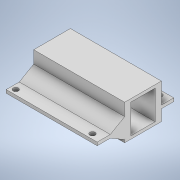
# Autodesk Inventor part: U2D2 Plate
Saved by Autodesk Inventor 2022 (Build 260153000, 153)
## iProperties
Created: 2021-09-20
Part Number: U2D2 Plate
Material: Generic
Document SubType Name: Modeling
Designer: kylem
Density: 1 g/cm^3
Appearance: Default
Author: kylem
Autodesk Inventor part; units mm, degrees
ref_plane "YZ Plane" through (0, 0, 0) normal (1, 0, 0) x (0, 1, 0)
ref_plane "XZ Plane" through (0, 0, 0) normal (0, 1, 0) x (-1, 0, 0)
sketch "Sketch1" plane through (0, 0, 0) normal (0, 1, 0) x (-1, 0, 0)
  line L0 (0, 0) -> (3, 0)
  line L1 (3, 0) -> (3, -3)
  line L2 (0, 0) -> (-48.04, 0)
  line L3 (-48.04, 0) -> (-54, 0)
  line L4 (3, -3) -> (-54, -3)
  line L5 (-54, -3) -> (-54, 45)
  line L6 (-54, 45) -> (3, 45)
  line L7 (3, 45) -> (3, -3)
  line L8 (3, 21) -> (6.1215, 21)
  circle A0 centre (0, 0) radius 1.65
  circle A1 centre (-48.04, 0) radius 1.65
  line L9 (0, 42) -> (-48.04, 42)
  circle A2 centre (0, 42) radius 1.65
  circle A3 centre (-48.04, 42) radius 1.65
  line L10 (-54, -3) -> (-54, 8.785)
  line L11 (-54, 8.785) -> (-9.9, 8.785)
  line L12 (-9.9, 8.785) -> (-9.9, 23.785)
  line L13 (-9.9, 23.785) -> (-54, 23.785)
  dimension "d0" = 3
  dimension "d1" = 3
  dimension "d2" = 48.04
  dimension "d3" = 5.96
  dimension "d4" = 48
  dimension "d5" = 3.3
  dimension "d6" = 3.3
  dimension "d7" = 11.785
  dimension "d8" = 44.1
  dimension "d9" = 15
  constraints: 28 end point, 5 perpendicular, 4 centre point, 4 coincident, 4 horizontal, 4 symmetric about line, 3 point on line, 2 parallel, 1 midpoint, 2 other
  measures "d0" distance of L0.start L0.end
  measures "d1" distance of L0.end L1.end
  measures "d2" distance of L0.start L2.end
  measures "d3" distance of L2.end L3.end
  measures "d4" distance of L4.end L5.end
  measures "d5" diameter of A0
  measures "d6" diameter of A1
  measures "d7" distance of L4.end L10.end
  measures "d8" distance of L10.end L11.end
  measures "d9" distance of L11.end L12.end
extrude "Extrusion1" add sketch "Sketch1" along normal blind 2 contours A0 L2 A1 L3 L5 L11 L12 L13 L6 L7 L0 | L0 L1 L4 L5 L3 A1 L2 A0
sketch "Sketch2" plane through (0, 0, 0) normal (0, -1, 0) x (1, 0, 0)
  line L0 (-3, -3) -> (-3, 45) projected
  line L1 (-3, -3) -> (-3, 5)
  line L2 (54, 8.785) -> (54, -3) projected
  line L3 (9.9, 8.785) -> (54, 8.785) projected
  line L4 (54, 8.785) -> (54, 4.785)
  line L5 (54, 8.785) -> (54, -3) projected
  line L6 (54, 23.785) -> (54, 27.785)
  line L7 (54, 45) -> (54, 23.785) projected
  line L8 (54, 27.785) -> (-3, 27.785)
  line L9 (-3, 5) -> (-3, 27.785)
  line L10 (9.9, 8.785) -> (54, 8.785) projected
  line L11 (54, 8.785) -> (9.9, 8.785)
  line L12 (9.9, 23.785) -> (9.9, 8.785) projected
  line L13 (9.9, 8.785) -> (9.9, 23.785)
  line L14 (9.9, 23.785) -> (54, 23.785)
  line L15 (-3, 5) -> (-3, 27.785)
  line L16 (-3, 27.785) -> (54, 27.785)
  line L17 (54, 27.785) -> (54, 4.785)
  line L18 (54, 4.785) -> (-3, 4.785)
  line L19 (-3, 4.785) -> (-3, 27.785)
  point P0 (0, 0)
  point P1 (-3, 4.785)
  dimension "d12" = 8
  dimension "d13" = 4
  dimension "d14" = 4
  constraints: 26 end point, 4 collinear, 4 point on line, 3 perpendicular, 2 parallel, 1 horizontal
  measures "d12" distance of L0.start L1.end
  measures "d13" distance of L2.start L4.end
  measures "d14" distance of L6.start L6.end
ref_plane "Work Plane1" through (0, -7, 0) normal (0, -1, 0) x (1, 0, 0)
sketch "Sketch4" plane through (54, 0, -3) normal (1, 0, 0) x (0, 0, -1)
  line L0 (-7.785, 0) -> (-7.785, -7) projected
  line L1 (-7.785, 0) -> (-7.785, 2)
  line L2 (0, 2) -> (-48, 2) projected
  line L3 (-7.785, 2) -> (-7.785, 15)
  line L4 (-30.785, 0) -> (-30.785, -7) projected
  line L5 (-30.785, 0) -> (-30.785, 15)
  line L6 (-7.785, 15) -> (-30.785, 15)
  line L7 (-26.785, -5) -> (-11.785, -5) projected
  line L8 (-11.785, 0) -> (-11.785, 2) projected
  line L9 (-11.785, -5) -> (-11.785, 2)
  line L10 (-11.785, 2) -> (-11.785, 13)
  line L11 (-26.785, 0) -> (-26.785, 2) projected
  line L12 (-26.785, 2) -> (-26.785, 13)
  line L13 (-26.785, 13) -> (-11.785, 13)
  point P0 (-3, 0)
  point P1 (-30.785, 2)
  dimension "d19" = 13
  dimension "d20" = 15
  dimension "d21" = 11
  dimension "d22" = 11
  constraints: 16 end point, 3 point on line, 2 collinear, 2 vertical
  measures "d19" distance of L1.end L3.end
  measures "d20" distance of L4.start L5.end
  measures "d21" distance of L8.end L10.end
  measures "d22" distance of L11.end L12.end
extrude "Extrusion5" add sketch "Sketch2" along normal blind 7 contours L0 L8 L6 L14 L12 L3 L2 L18
sketch "Sketch5" plane through (0, -7, 0) normal (0, -1, 0) x (1, 0, 0)
  line L0 (9.9, 23.785) -> (54, 23.785) projected
  line L1 (54, 23.785) -> (9.9, 23.785)
  line L2 (9.9, 23.785) -> (9.9, 8.785)
  line L3 (9.9, 8.785) -> (54, 8.785)
  line L4 (54, 8.785) -> (54, 23.785)
  point P0 (0, 0)
  constraints: 8 end point, 2 parallel, 1 horizontal, 1 perpendicular
extrude "Extrusion6" add sketch "Sketch5" against normal blind 2
extrude "Extrusion7" add sketch "Sketch4" against normal blind 44.1 contours L2 L10 L13 L12 L5 L6 L3
sketch "Sketch6" plane through (9.9, 0, -3) normal (-1, 0, 0) x (0, 0, 1)
  line L0 (7.785, 15) -> (7.785, 2) projected
  line L1 (48, 2) -> (30.785, 2) projected
  line L2 (7.785, 15) -> (30.785, 15)
  line L3 (30.785, 15) -> (30.785, 2)
  line L4 (30.785, 2) -> (7.785, 2)
  line L5 (7.785, 2) -> (7.785, 15)
  point P0 (3, 0)
  constraints: 8 end point, 2 parallel, 1 horizontal, 1 perpendicular
extrude "Extrusion8" add sketch "Sketch6" along normal blind 12.9
sketch "Sketch8" plane through (9.9, -5, 8.785) normal (0, 0, 1) x (1, 0, 0)
  line L0 (44.1, 0) -> (44.1, 18) projected
  line L1 (44.1, 0) -> (18.5, 0)
  line L2 (0, 0) -> (44.1, 0) projected
  line L3 (18.5, 0) -> (5.5, 0)
  line L4 (5.5, 0) -> (5.5, 1)
  line L5 (-12.9, 5) -> (44.1, 5) projected
  line L6 (5.5, 1) -> (14.6, 1)
  line L7 (44.1, -2) -> (-12.9, -2) projected
  line L8 (44.1, 18) -> (0, 18) projected
  line L9 (14.6, -2) -> (36.6, -2) construction
  line L10 (5.5, 1) -> (5.5, 18)
  line L11 (5.5, 18) -> (14.6, 18)
  line L12 (44.1, 18) -> (0, 18) projected
  line L13 (5.5, 1) -> (5.5, 17)
  line L14 (5.5, 17) -> (14.6, 17)
  line L15 (5.5, 17) -> (18.5, 17)
  line L16 (18.5, 17) -> (18.5, 1)
  line L17 (18.5, 1) -> (5.5, 1)
  point P0 (-9.9, 5)
  point P1 (5.5, 5)
  point P2 (14.6, 1)
  dimension "d33" = 25.6
  dimension "d34" = 13
  dimension "d35" = 1
  dimension "d39" = 16
  dimension "d42" = 13
  constraints: 24 end point, 7 point on line, 3 perpendicular, 1 collinear, 1 horizontal
  measures "d33" distance of L0.start L1.end
  measures "d34" distance of L1.end L3.end
  measures "d35" distance of L3.end L4.end
  measures "d39" distance of L4.end L13.end
  measures "d42" distance of L13.end L15.end
extrude "Extrusion10" cut sketch "Sketch8" against normal blind 12.9 contours L16 L17 L6 L10 L5 | L5 L10 L14 L15 L16
sketch "Sketch11" plane through (0, 2, 0) normal (0, 1, 0) x (1, 0, 0)
  circle A0 centre (48.04, 0) radius 1.65 projected
  circle A1 centre (0, 0) radius 1.65 projected
  line L0 (48.04, 0) -> (0, 0)
  line L1 (24.02, 0) -> (24.02, 5.2317)
  line L2 (24.02, 0) -> (10.02, 0)
  line L3 (10.02, 0) -> (38.02, 0)
  line L4 (38.02, 0) -> (38.02, 7.5339)
  line L5 (54, -4.785) -> (-3, -4.785) projected
  line L6 (38.02, 7.5339) -> (10.02, 7.5339)
  line L7 (10.02, 7.5339) -> (10.02, -4.785)
  line L8 (10.02, -4.785) -> (38.02, -4.785)
  line L9 (38.02, -4.785) -> (38.02, 7.5339)
  dimension "d74" = 14
  dimension "d75" = 28
  constraints: 18 end point, 3 point on line, 2 horizontal, 2 parallel, 2 perpendicular, 1 midpoint, 1 vertical
  measures "d74" distance of L1.start L2.end
  measures "d75" distance of L2.end L3.end
extrude "Extrusion12" cut sketch "Sketch11" against normal blind 10 contours L9 L5 L7 L0 | L0 L7 L6 L4
chamfer "Chamfer9" distance 7.785 angle 45 2 edges at (38.02, 1, -3) (10.02, 1, -3)
sketch "Sketch12" plane through (54, 13, 8.785) normal (0, -1, 0) x (1, 0, 0)
  line L0 (0, 0) -> (-44.1, 0) projected
  line L1 (-44.1, 0) -> (-44.1, 15) projected
  line L2 (0, 0) -> (-44.1, 0)
  line L3 (-44.1, 0) -> (-44.1, 15)
  line L4 (-44.1, 15) -> (0, 15)
  line L5 (0, 15) -> (0, 0)
  point P0 (-54, -8.785)
  constraints: 8 end point, 2 parallel, 1 horizontal, 1 perpendicular
extrude "Extrusion13" cut sketch "Sketch12" against normal blind 0.125
sketch "Sketch13" plane through (0, -5, 0) normal (0, 1, 0) x (1, 0, 0)
  line L0 (54, -23.785) -> (9.9, -23.785) projected
  line L1 (9.9, -8.785) -> (54, -8.785)
  line L2 (54, -8.785) -> (54, -23.785)
  line L3 (54, -23.785) -> (9.9, -23.785)
  line L4 (9.9, -23.785) -> (9.9, -8.785)
  point P0 (0, 0)
  constraints: 8 end point, 2 parallel, 1 horizontal, 1 perpendicular
extrude "Extrusion14" cut sketch "Sketch13" against normal blind 0.125
sketch "Sketch14" plane through (54, 13.125, 23.785) normal (0, 0, -1) x (-1, 0, 0)
  line L0 (44.1, -18.25) -> (44.1, 0) projected
  line L1 (0, -18.25) -> (44.1, -18.25) projected
  line L2 (44.1, 0) -> (0, 0)
  line L3 (0, 0) -> (0, -18.25)
  line L4 (0, -18.25) -> (44.1, -18.25)
  line L5 (44.1, -18.25) -> (44.1, 0)
  point P0 (54, -13.125)
  constraints: 8 end point, 2 parallel, 1 horizontal, 1 perpendicular
extrude "Extrusion15" cut sketch "Sketch14" against normal blind 0.05
sketch "Sketch15" plane through (9.9, 13.125, 8.785) normal (0, 0, 1) x (1, 0, 0)
  line L0 (44.1, 0) -> (0, 0) projected
  line L1 (44.1, 0) -> (44.1, -18.25) projected
  line L2 (0, 0) -> (44.1, 0)
  line L3 (44.1, 0) -> (44.1, -18.25)
  line L4 (44.1, -18.25) -> (0, -18.25)
  line L5 (0, -18.25) -> (0, 0)
  point P0 (-9.9, -13.125)
  constraints: 8 end point, 2 parallel, 1 horizontal, 1 perpendicular
extrude "Extrusion16" cut sketch "Sketch15" against normal blind 0.05
chamfer "Chamfer12" distance 9 angle 30 1 edges at (25.5, 2, 27.785) measured on face at (32.6017, 2, 32.1586)
chamfer "Chamfer13" distance 9 angle 30 1 edges at (25.5, 0, 27.785) measured on face at (32.6017, 0, 32.1586)
body "Solid1"
